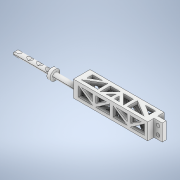
# Autodesk Inventor part: Final design part 2
Saved by Autodesk Inventor 2021 (Build 250183000, 183)
## iProperties
Created: 2021-03-23
Part Number: Final design part 2
Material: ABS Plastic
Document SubType Name: Modeling
Designer: kcf23
Density: 1.06 g/cm^3
Appearance: Smooth - White
Mass: 30.8372 g
Surface Area: 218.207 cm^2
Volume: 30.8372 cm^3
Author: kcf23
Autodesk Inventor part; units mm, degrees
ref_plane "YZ Plane" through (0, 0, 0) normal (1, 0, 0) x (0, 1, 0)
ref_plane "XZ Plane" through (0, 0, 0) normal (0, 1, 0) x (-1, 0, 0)
ref_plane "XY Plane" through (0, 0, 0) normal (0, 0, 1) x (1, 0, 0)
sketch "Sketch1" plane through (0, 0, 0) normal (0, 0, 1) x (1, 0, 0)
  line L0 (0, 0) -> (127, 0)
  line L1 (127, 0) -> (127, 25.4)
  line L2 (127, 25.4) -> (0, 25.4)
  line L3 (0, 25.4) -> (0, 0)
  line L4 (114.3, 0) -> (114.3, 25.4)
  line L5 (109.22, 5.08) -> (109.22, 20.32)
  line L6 (109.22, 5.08) -> (87.63, 5.08)
  line L7 (87.63, 5.08) -> (109.22, 20.32)
  line L8 (82.55, 5.08) -> (60.96, 5.08)
  line L9 (60.96, 5.08) -> (60.96, 20.32)
  line L10 (60.96, 20.32) -> (82.55, 5.08)
  line L11 (55.88, 5.08) -> (55.88, 20.32)
  line L12 (55.88, 5.08) -> (34.29, 5.08)
  line L13 (34.29, 5.08) -> (55.88, 20.32)
  line L14 (29.21, 5.08) -> (7.62, 5.08)
  line L15 (7.62, 5.08) -> (7.62, 20.32)
  line L16 (7.62, 20.32) -> (29.21, 5.08)
  line L17 (87.63, 10.16) -> (87.63, 20.32)
  line L18 (87.63, 20.32) -> (104.14, 20.32)
  line L19 (104.14, 20.32) -> (87.63, 10.16)
  line L20 (66.04, 20.32) -> (82.55, 20.32)
  line L21 (82.55, 20.32) -> (82.55, 10.16)
  line L22 (82.55, 10.16) -> (66.04, 20.32)
  line L23 (50.8, 20.32) -> (34.29, 20.32)
  line L24 (34.29, 20.32) -> (34.29, 10.16)
  line L25 (34.29, 10.16) -> (50.8, 20.32)
  line L26 (29.21, 10.16) -> (29.21, 20.32)
  line L27 (29.21, 20.32) -> (12.7, 20.32)
  line L28 (12.7, 20.32) -> (29.21, 10.16)
  line L29 (120.65, 25.4) -> (120.65, 0)
  circle A0 centre (120.65, 19.05) radius 2.7432
  circle A1 centre (120.65, 6.35) radius 2.7432
  dimension "d0" = 127
  dimension "d1" = 25.4
  dimension "d3" = 12.7
  dimension "d4" = 15.24
  dimension "d5" = 21.59
  dimension "d6" = 21.59
  dimension "d7" = 21.59
  dimension "d8" = 21.59
  dimension "d9" = 16.51
  dimension "d10" = 16.51
  dimension "d63" = 5.08
  dimension "d64" = 5.08
  dimension "d100" = 5.4864
  dimension "d101" = 5.4864
  constraints: 60 end point, 12 point on line, 7 perpendicular, 5 horizontal, 4 parallel, 3 vertical, 2 centre point, 2 coincident
  measures "d0" distance of L2.end L1.end
  measures "d1" distance of L1.end L0.end
  measures "d3" distance between parallel lines of L1 L4
  measures "d4" distance of L5.start L5.end
  measures "d5" distance of L5.start L6.end
  measures "d6" distance of L8.start L8.end
  measures "d7" distance of L11.start L12.end
  measures "d8" distance of L14.start L14.end
  measures "d9" distance of L17.end L18.end
  measures "d10" distance of L26.end L27.end
  measures "d63" distance between parallel lines of L27 L2
  measures "d64" distance between parallel lines of L0 L14
  measures "d100" diameter of A0
  measures "d101" diameter of A1
extrude "Extrusion1" add sketch "Sketch1" along normal blind 25.4
sketch "Sketch3" plane through (0, 25.4, 0) normal (0, 1, 0) x (1, 0, 0)
  line L0 (127, -25.4) -> (0, -25.4) projected
  line L1 (127, 0) -> (0, 0) projected
  line L2 (0, 0) -> (0, -25.4) projected
  line L3 (0, -25.4) -> (127, -25.4) projected
  line L4 (0, 0) -> (5.08, 0)
  line L5 (5.08, 0) -> (5.08, -25.4)
  line L6 (5.08, -25.4) -> (0, -25.4)
  line L7 (0, -25.4) -> (0, 0)
  line L8 (127, 0) -> (121.92, 0)
  line L9 (121.92, 0) -> (121.92, -25.4)
  line L10 (121.92, -25.4) -> (127, -25.4)
  line L11 (127, -25.4) -> (127, 0)
  line L12 (5.08, 0) -> (121.92, 0)
  line L13 (121.92, 0) -> (121.92, -5.08)
  line L14 (121.92, -5.08) -> (5.08, -5.08)
  line L15 (5.08, -5.08) -> (5.08, 0)
  line L16 (121.92, -25.4) -> (5.08, -25.4)
  line L17 (5.08, -25.4) -> (5.08, -20.32)
  line L18 (5.08, -20.32) -> (121.92, -20.32)
  line L19 (121.92, -20.32) -> (121.92, -25.4)
  line L20 (127, 0) -> (127, -25.4) projected
  line L21 (127, -12.7) -> (114.3, -12.7)
  line L22 (127, -15.748) -> (114.3, -15.748)
  line L23 (114.3, -15.748) -> (114.3, -9.652)
  line L24 (114.3, -9.652) -> (127, -9.652)
  line L25 (127, -9.652) -> (127, -15.748)
  line L26 (127, -15.748) -> (114.3, -9.652) construction
  line L27 (114.3, -15.748) -> (127, -9.652) construction
  line L28 (114.3, -25.4) -> (114.3, 0)
  line L29 (0, 0) -> (127, 0) projected
  line L30 (114.3, -9.652) -> (127, -9.652)
  line L31 (127, -15.748) -> (114.3, -15.748)
  point P0 (109.22, -25.4)
  point P1 (120.65, -12.7)
  point P2 (121.92, -9.652)
  dimension "d13" = 25.4
  dimension "d14" = 5.08
  dimension "d15" = 5.08
  dimension "d16" = 5.08
  dimension "d17" = 5.08
  dimension "d18" = 17.78
  dimension "d19" = 12.7
  dimension "d20" = 6.096
  constraints: 52 end point, 11 equal length, 7 perpendicular, 6 horizontal, 6 point on line, 4 midpoint
  measures "d13" distance between parallel lines of L0 L1
  measures "d14" distance of L5.end L6.end
  measures "d15" distance of L10.end L9.end
  measures "d16" distance of L12.end L13.end
  measures "d17" distance of L16.end L17.end
  measures "d18" distance of L0.start point (109.22, -25.4)
  measures "d19" distance of L21.start L21.end
  measures "d20" distance of L22.end L23.end
extrude "Extrusion2" cut sketch "Sketch3" against normal blind 25.4 contours L0 L9 L22 L11 | L0 L28 L18 L9 | L18 L28 L22 L9 | L24 L9 L1 L11 | L24 L28 L14 L9 | L9 L14 L28 L1
sketch "Sketch4" plane through (0, 25.4, 25.4) normal (0, 1, 0) x (1, 0, 0)
  line L0 (127, 0) -> (127, 25.4)
  line L1 (127, 25.4) -> (0, 25.4)
  line L2 (0, 25.4) -> (0, 0)
  line L3 (7.0215, 5.08) -> (32.4215, 5.08)
  line L4 (32.4215, 5.08) -> (32.4215, 20.32)
  line L5 (32.4215, 20.32) -> (7.0215, 5.08)
  line L6 (37.5015, 3.81) -> (37.5015, 19.05)
  line L7 (37.5015, 19.05) -> (52.7415, 19.05)
  line L8 (52.7415, 19.05) -> (37.5015, 3.81)
  line L9 (57.8215, 19.05) -> (73.0615, 19.05)
  line L10 (73.0615, 19.05) -> (73.0615, 3.81)
  line L11 (73.0615, 3.81) -> (57.8215, 19.05)
  line L12 (78.1415, 20.32) -> (78.1415, 5.08)
  line L13 (78.1415, 5.08) -> (103.5415, 5.08)
  line L14 (103.5415, 5.08) -> (78.1415, 20.32)
  line L15 (9.048, 20.32) -> (9.048, 11.8849)
  line L16 (9.048, 20.32) -> (24.288, 20.32)
  line L17 (24.288, 20.32) -> (9.048, 11.8849)
  line L18 (45.1215, 5.08) -> (52.7415, 5.08)
  line L19 (52.7415, 5.08) -> (52.7415, 12.7)
  line L20 (52.7415, 12.7) -> (45.1215, 5.08)
  line L21 (57.8215, 5.08) -> (57.8215, 12.7)
  line L22 (57.8215, 5.08) -> (65.4415, 5.08)
  line L23 (65.4415, 5.08) -> (57.8215, 12.7)
  line L24 (105.8158, 10.4367) -> (105.8158, 20.32)
  line L25 (105.8158, 20.32) -> (90.5758, 20.32)
  line L26 (90.5758, 20.32) -> (105.8158, 10.4367)
  line L27 (0, 0) -> (127, 0)
  line L28 (114.3, 0) -> (0, 0) projected
  point P0 (0, 25.4)
  point P1 (26.0715, 5.08)
  dimension "d40" = 127
  dimension "d41" = 25.4
  dimension "d42" = 25.4
  dimension "d43" = 15.24
  dimension "d44" = 15.24
  dimension "d45" = 15.24
  dimension "d46" = 15.24
  dimension "d47" = 25.4
  dimension "d48" = 15.24
  dimension "d49" = 7.62
  dimension "d50" = 7.62
  dimension "d51" = 15.24
  dimension "d52" = 2
  dimension "d53" = 2
  dimension "d65" = 5.08
  dimension "d66" = 5.08
  dimension "d67" = 5.08
  dimension "d68" = 5.08
  dimension "d69" = 6.35
  dimension "d70" = 5.08
  dimension "d71" = 5.08
  constraints: 56 end point, 9 perpendicular, 4 point on line, 4 vertical, 3 horizontal, 1 parallel
  measures "d40" distance of L1.end L0.end
  measures "d41" distance of L0.start L0.end
  measures "d42" distance of L3.start L3.end
  measures "d43" distance of L3.end L4.end
  measures "d44" distance of L6.end L7.end
  measures "d45" distance of L9.start L9.end
  measures "d46" distance of L9.end L10.end
  measures "d47" distance of L12.end L13.end
  measures "d48" distance of L15.start L16.end
  measures "d49" distance of L18.end L19.end
  measures "d50" distance of L21.start L22.end
  measures "d51" distance of L24.end L25.end
  measures "d52" angle of L14 L26
  measures "d53" angle of L5 L17
  measures "d65" distance between parallel lines of L16 L1
  measures "d66" distance between parallel lines of L28 L3
  measures "d67" distance between parallel lines of L28 L13
  measures "d68" distance between parallel lines of L25 L1
  measures "d69" distance between parallel lines of L7 L1
  measures "d70" distance between parallel lines of L27 L18
  measures "d71" distance from line of L1 L12.start
extrude "Extrusion3" cut sketch "Sketch4" against normal blind 25.4 contours L5 L4 L3 | L6 L7 L8 | L9 L10 L11 | L14 L13 L12 | L16 L17 L15 | L20 L19 L18 | L21 L23 L22 | L26 L25 L24
sketch "Sketch5" plane through (0, 0, 0) normal (-1, 0, 0) x (0, 0, 1)
  line L0 (20.32, 5.08) -> (5.08, 5.08)
  line L1 (5.08, 5.08) -> (5.08, 20.32)
  line L2 (5.08, 20.32) -> (20.32, 20.32)
  line L3 (20.32, 20.32) -> (20.32, 5.08)
  line L4 (0, 0) -> (25.4, 0) projected
  line L5 (0, 25.4) -> (25.4, 25.4) projected
  line L6 (25.4, 25.4) -> (25.4, 0) projected
  line L7 (0, 25.4) -> (0, 0) projected
  dimension "d57" = 5.08
  dimension "d58" = 5.08
  dimension "d59" = 5.08
  dimension "d60" = 5.08
  constraints: 8 end point, 2 parallel, 1 horizontal, 1 perpendicular
  measures "d57" distance between parallel lines of L4 L0
  measures "d58" distance between parallel lines of L5 L2
  measures "d59" distance between parallel lines of L3 L6
  measures "d60" distance between parallel lines of L7 L1
extrude "Extrusion4" cut sketch "Sketch5" against normal blind 112.7125 contours L0 L1 L2 L3
sketch "Sketch8" plane through (0, 0, 0) normal (0, -1, 0) x (1, 0, 0)
  point P0 (0, 0)
sketch "Sketch9" plane through (0, 0, 0) normal (-1, 0, 0) x (0, 0, 1)
  line L0 (20.32, 0) -> (5.08, 0) projected
  line L1 (16.5088, 7.62) -> (8.8912, 7.62)
  line L2 (8.8912, 7.62) -> (8.8912, 0)
  line L3 (8.8912, 0) -> (16.5088, 0)
  line L4 (16.5088, 0) -> (16.5088, 7.62)
  line L5 (12.7, 5.08) -> (12.7, 0) projected
  line L6 (16.5088, 7.62) -> (8.8912, 0) construction
  line L7 (8.8912, 7.62) -> (16.5088, 0) construction
  point P0 (0, 0)
  point P1 (12.7, 3.81)
  constraints: 12 end point, 2 midpoint, 2 parallel, 2 point on line, 1 horizontal, 1 perpendicular
extrude "Extrusion7" add sketch "Sketch9" along normal blind 101.6
sketch "Sketch10" plane through (0, 5.08, 8.8912) normal (0, 0, -1) x (-1, 0, 0)
  line L0 (101.6, 2.54) -> (101.6, -5.08) projected
  line L1 (101.6, 0.5132) -> (92.1889, 2.54)
  line L2 (0, 2.54) -> (101.6, 2.54) projected
  line L3 (101.6, -2.8231) -> (92.1889, -5.08)
  line L4 (0, -5.08) -> (101.6, -5.08) projected
  line L5 (83.8482, 2.54) -> (79.1901, 0.5132)
  line L6 (79.1901, 0.5132) -> (74.5319, 2.54)
  line L7 (69.4436, 2.54) -> (64.6204, 0.9452)
  line L8 (64.6204, 0.9452) -> (59.7973, 2.54)
  line L9 (59.7973, 2.54) -> (54.7173, 2.54)
  line L10 (54.7173, 2.54) -> (50.3147, 0.0055)
  line L11 (50.3147, 0.0055) -> (45.774, 2.54)
  dimension "d80" = 5.08
  dimension "d81" = 5.08
  dimension "d82" = 5.08
  dimension "d83" = 5.08
  dimension "d84" = 5.08
  dimension "d85" = 5.08
  dimension "d86" = 55.826
  constraints: 18 end point, 7 point on line
  measures "d80" distance of L5.start L5.end
  measures "d81" distance of L5.end L6.end
  measures "d82" distance of L7.start L7.end
  measures "d83" distance of L7.end L8.end
  measures "d84" distance of L8.end L9.end
  measures "d85" distance of L9.end L10.end
  measures "d86" horizontal distance of L11.end L0.end
extrude "Extrusion8" cut sketch "Sketch10" against normal blind 101.6
sketch "Sketch11" plane through (-101.6, 0, 0) normal (-1, 0, 0) x (0, 0, 1)
  line L0 (12.7, 25.4) -> (12.7, 0) projected
  circle A0 centre (12.7, 3.81) radius 3.81
  line L1 (16.5088, 7.62) -> (8.8912, 7.62) projected
  line L2 (19.5843, -3.2588) -> (5.8157, -3.2588)
  line L3 (5.8157, -3.2588) -> (5.8157, 10.8788)
  line L4 (5.8157, 10.8788) -> (19.5843, 10.8788)
  line L5 (19.5843, 10.8788) -> (19.5843, -3.2588)
  line L6 (19.5843, -3.2588) -> (5.8157, 10.8788) construction
  line L7 (5.8157, -3.2588) -> (19.5843, 10.8788) construction
  point P0 (0, 0)
  point P1 (12.7, 5.08)
  constraints: 12 end point, 2 midpoint, 2 parallel, 1 centre point, 1 horizontal, 1 perpendicular, 1 point on line, 1 tangent
sketch "Sketch12" plane through (0, 7.62, 16.5088) normal (0, 1, 0) x (1, 0, 0)
  line L0 (0, 0) -> (-92.1889, 0) projected
  line L1 (0, 7.6175) -> (-45.774, 7.6175) projected
  line L2 (-46.0944, 0) -> (-43.5544, 0)
  line L3 (-43.5544, 0) -> (-43.5544, 7.6175)
  line L4 (-43.5544, 7.6175) -> (-46.0944, 7.6175)
  line L5 (-46.0944, 7.6175) -> (-46.0944, 0)
  point P0 (0, 16.5088)
  dimension "d89" = 2.54
  constraints: 8 end point, 2 parallel, 1 horizontal, 1 midpoint, 1 perpendicular, 1 point on line
  measures "d89" distance of L4.end L3.end
extrude "Extrusion9" add sketch "Sketch12" along normal blind 15.24
extrude "Extrusion10" cut sketch "Sketch11" against normal blind 101.6
sketch "Sketch13" plane through (-46.0944, 22.86, 8.8912) normal (-1, 0, 0) x (0, 0, 1)
  line L0 (3.8088, 2.54) -> (3.8088, -22.86) projected
  circle A0 centre (3.8088, -19.05) radius 7.62
  point P0 (-8.8912, -22.86)
  point P1 (3.8088, -17.78)
  dimension "d94" = 15.24
  constraints: 1 centre point, 1 point on line
  measures "d94" diameter of A0
extrude "Extrusion11" add sketch "Sketch13" against normal blind 5.08
sketch "Sketch14" plane through (-101.6, 0, 0) normal (-1, 0, 0) x (0, 0, 1)
  line L0 (12.7, 25.4) -> (12.7, 0) projected
  circle A0 centre (12.7, 3.81) radius 7.62
  circle A1 centre (12.7, 3.81) radius 21.733
  point P0 (0, 0)
  point P1 (12.7, 5.08)
  dimension "d97" = 15.24
  constraints: 2 centre point, 1 coincident, 1 point on line
  measures "d97" diameter of A0
extrude "Extrusion12" cut sketch "Sketch14" against normal blind 101.6
sketch "Sketch15" plane through (114.3, 25.4, 15.748) normal (0, 0, 1) x (1, 0, 0)
  circle A0 centre (6.35, -19.05) radius 2.7432
  circle A1 centre (6.35, -6.35) radius 2.7432
  point P0 (-114.3, -25.4)
  dimension "d102" = 5.4864
  dimension "d103" = 5.4864
  constraints: 2 centre point
  measures "d102" diameter of A0
  measures "d103" diameter of A1
extrude "Extrusion13" cut sketch "Sketch15" against normal blind 25.4
body "Solid1"
